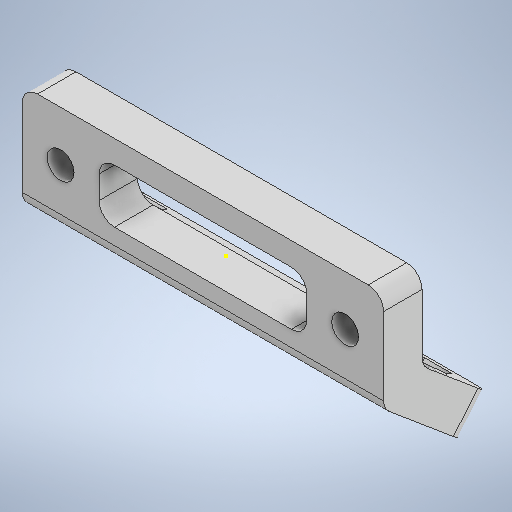
# Autodesk Inventor part: Part3
Saved by Autodesk Inventor 2025.1 (Build 291241000, 241)
## iProperties
Created: 2024-09-08
Part Number: Part3
Material: 一般
Document SubType Name: Modeling
Designer: right
Density: 1 g/cm^3
Appearance: 既定
Author: right
Autodesk Inventor part; units mm, degrees
ref_plane "YZ Plane" through (0, 0, 0) normal (1, 0, 0) x (0, 1, 0)
ref_plane "XZ Plane" through (0, 0, 0) normal (0, 1, 0) x (-1, 0, 0)
ref_plane "XY Plane" through (0, 0, 0) normal (0, 0, 1) x (1, 0, 0)
sketch "スケッチ1" plane through (0, 0, 0) normal (0, 0, 1) x (1, 0, 0)
  circle A0 centre (-18.5, 0) radius 1.75
  circle A1 centre (18.5, 0) radius 1.75
  circle A2 centre (-18.5, 0) radius 5
  circle A3 centre (18.5, 0) radius 5
  line L0 (-23.5, 6.5) -> (23.5, 6.5)
  line L1 (23.5, 6.5) -> (23.5, -6.5)
  line L2 (23.5, -6.5) -> (-23.5, -6.5)
  line L3 (-23.5, -6.5) -> (-23.5, 6.5)
  point P0 (0, 0)
  point P1 (-23.5, 0)
  dimension "d0" = 3.5
  dimension "d1" = 3.5
  dimension "d2" = 37
  dimension "d3" = 18.5
  dimension "d4" = 10
  dimension "d5" = 10
  dimension "d6" = 13
  constraints: 8 end point, 4 centre point, 3 horizontal alignment, 2 coincident, 2 parallel, 2 tangent, 1 horizontal, 1 midpoint, 1 perpendicular
  measures "d0" diameter of A0
  measures "d1" diameter of A1
  measures "d2" distance of A1.centre A0.centre
  measures "d3" distance of point (0, 0) A0.centre
  measures "d4" diameter of A2
  measures "d5" diameter of A3
  measures "d6" distance of L2.end L0.start
extrude "押し出し1" add sketch "スケッチ1" along normal blind 5 contours A2 | A3 | L3 L0 L1 L2
sketch "スケッチ2" plane through (0, 0, 5) normal (0, 0, 1) x (1, 0, 0)
  line L0 (-13.5, -3.5) -> (13.5, -3.5)
  line L1 (13.5, -3.5) -> (13.5, 3.5)
  line L2 (13.5, 3.5) -> (-13.5, 3.5)
  line L3 (-13.5, 3.5) -> (-13.5, -3.5)
  line L4 (-13.5, -3.5) -> (13.5, 3.5) construction
  line L5 (13.5, -3.5) -> (-13.5, 3.5) construction
  line L6 (23.5, 6.5) -> (-23.5, 6.5) projected
  circle A0 centre (-18.5, 0) radius 1.75 projected
  point P0 (0, 0)
  dimension "d9" = 3
  dimension "d10" = 5
  constraints: 12 end point, 2 midpoint, 2 parallel, 1 horizontal, 1 perpendicular
  measures "d9" distance between parallel lines of L6 L2
  measures "d10" distance from line of A0.centre L3
extrude "押し出し2" cut sketch "スケッチ2" against normal through all contours L3 L2 L1 L0
sketch "スケッチ3" plane through (0, 0, 0) normal (0, 0, -1) x (-1, 0, 0)
  circle A0 centre (-18.5, 0) radius 1.75 construction
  circle A1 centre (-18.5, 0) radius 3 construction
  line L0 (-20.2321, 3) -> (-16.7679, 3)
  line L1 (-21.9641, 0) -> (-20.2321, 3)
  line L2 (-20.2321, -3) -> (-21.9641, 0)
  line L3 (-16.7679, -3) -> (-20.2321, -3)
  line L4 (-15.0359, 0) -> (-16.7679, -3)
  line L5 (-16.7679, 3) -> (-15.0359, 0)
  line L6 (-23.5, 6.5) -> (23.5, 6.5) construction
  line L7 (0, 6.5) -> (0, 0) construction
  circle A2 centre (18.5, 0) radius 1.75 construction
  circle A3 centre (18.5, 0) radius 3 construction
  line L8 (20.2321, 3) -> (16.7679, 3)
  line L9 (21.9641, 0) -> (20.2321, 3)
  line L10 (20.2321, -3) -> (21.9641, 0)
  line L11 (16.7679, -3) -> (20.2321, -3)
  line L12 (15.0359, 0) -> (16.7679, -3)
  line L13 (16.7679, 3) -> (15.0359, 0)
  point P0 (-21.5, 6.5)
  point P1 (21.5, 6.5)
  dimension "d14" = 6
  dimension "d17" = 360
  constraints: 26 end point, 14 symmetric about line, 4 coincident, 3 centre point, 1 horizontal, 1 midpoint, 1 tangent, 1 vertical, 21 other
  measures "d14" diameter of A1
extrude "押し出し3" cut sketch "スケッチ3" against normal blind 2
sketch "スケッチ5" plane through (23.5, -6.5, 0) normal (1, 0, 0) x (0, 0, -1)
  line L0 (0, 0) -> (-5, 0) projected
  line L1 (-5, 0) -> (5.5946, -8.8899)
  line L2 (5.5946, -8.8899) -> (8.8085, -5.0597)
  line L3 (0, 0) -> (0, 13) projected
  line L4 (0, 2.3315) -> (8.8085, -5.0597)
  point P0 (0, 6.5)
  dimension "d27" = 5
  dimension "d28" = 130
  dimension "d29" = 10
  constraints: 6 end point, 1 parallel, 1 perpendicular, 1 point on line
  measures "d27" distance between parallel lines of L1 L4
  measures "d28" angle of L3 L4
  measures "d29" distance from line of L0.start L2
extrude "押し出し5" add sketch "スケッチ5" against normal up to surface (47 mm away)
fillet "フィレット2" radius 2 2 edges at (0, -6.5, 5) (0, -4.1685, 0)
sketch "スケッチ6" plane through (-23.5, -11.5597, -8.8085) normal (0, 0.7660444, -0.6427876) x (1, 0, 0)
  circle A0 centre (5, -5.283) radius 1.75
  line L0 (0, 0) -> (0, -10.5661) projected
  ellipse E0 centre (5, -15.7102) end of major axis (3.25, -15.7102) minor radius 1.1249 projected
  line L1 (47, -22.1865) -> (0, -22.1865) construction
  line L2 (23.5, -22.1865) -> (23.5, 0) construction
  line L3 (47, 0) -> (0, 0) construction
  circle A1 centre (42, -5.283) radius 1.75
  point P0 (23.5, -14.1781)
  point P1 (0, -5.283)
  dimension "d33" = 3.5
  constraints: 3 midpoint, 2 centre point, 2 end point, 1 horizontal alignment, 1 symmetric about line, 1 vertical alignment, 2 other
  measures "d33" diameter of A0
extrude "押し出し6" cut sketch "スケッチ6" against normal through all contours A0 | A1
fillet "フィレット3" radius 2 4 edges at (-13.5, -3.5, 2.4912) (-13.5, 3.5, 2.5) (13.5, 3.5, 2.5) (13.5, -3.5, 2.4912)
sketch "スケッチ7" plane through (-23.5, -11.5597, -8.8085) normal (0, 0.7660444, -0.6427876) x (1, 0, 0)
  circle A0 centre (42, -5.283) radius 1.75 projected
  circle A1 centre (42, -5.283) radius 3 construction
  line L0 (47, -22.1865) -> (0, -22.1865) construction
  line L1 (23.5, -22.1865) -> (23.5, 0) construction
  line L2 (47, 0) -> (0, 0) construction
  line L3 (43.7321, -8.283) -> (40.2679, -8.283)
  line L4 (45.4641, -5.283) -> (43.7321, -8.283)
  line L5 (43.7321, -2.283) -> (45.4641, -5.283)
  line L6 (40.2679, -2.283) -> (43.7321, -2.283)
  line L7 (38.5359, -5.283) -> (40.2679, -2.283)
  line L8 (40.2679, -8.283) -> (38.5359, -5.283)
  circle A2 centre (5, -5.283) radius 1.75
  circle A3 centre (5, -5.283) radius 3 construction
  line L9 (3.2679, -8.283) -> (6.7321, -8.283)
  line L10 (1.5359, -5.283) -> (3.2679, -8.283)
  line L11 (3.2679, -2.283) -> (1.5359, -5.283)
  line L12 (6.7321, -2.283) -> (3.2679, -2.283)
  line L13 (8.4641, -5.283) -> (6.7321, -2.283)
  line L14 (6.7321, -8.283) -> (8.4641, -5.283)
  point P0 (23.5, -14.1781)
  point P1 (6.7321, -8.283)
  point P2 (3.2679, -8.283)
  point P3 (43.7321, -8.283)
  point P4 (40.2679, -8.283)
  dimension "d37" = 6
  dimension "d40" = 360
  constraints: 26 end point, 14 symmetric about line, 4 coincident, 3 centre point, 2 midpoint, 1 horizontal, 1 tangent, 21 other
  measures "d37" diameter of A1
extrude "押し出し7" cut sketch "スケッチ7" against normal blind 2
fillet "フィレット4" radius 2 4 edges at (23.5, 6.5, 2.5) (23.5, -13.4748, -7.2015) (-23.5, -13.4748, -7.2015) (-23.5, 6.5, 2.5)
sketch "スケッチ8" plane through (-23.5, -4.7679, -0.7144) normal (0, 0.7660444, -0.6427876) x (1, 0, 0)
  point P0 (23.5, -3.6121)
equation "\"d1\" = d0"
equation "\"d3\" = 0.5 * d2"
equation "\"d5\" = d4"
